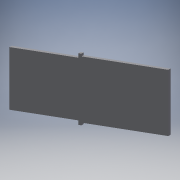
# Autodesk Inventor part: Zonnepaneel V5.0 print Versie
Saved by Autodesk Inventor 2018.3 (Build 223284000, 284)
## iProperties
Created: 2020-11-27
Part Number: Zonnepaneel V5.0 print Versie
Material: Generic
Document SubType Name: Modeling
Designer: daanv
Density: 1 g/cm^3
Appearance: Default
Author: daanv
Autodesk Inventor part; units mm, degrees
ref_plane "YZ Plane" through (0, 0, 0) normal (1, 0, 0) x (0, 1, 0)
ref_plane "XZ Plane" through (0, 0, 0) normal (0, 1, 0) x (-1, 0, 0)
ref_plane "XY Plane" through (0, 0, 0) normal (0, 0, 1) x (1, 0, 0)
sketch "Sketch6" plane through (0, 0, 0) normal (0, 0, 1) x (1, 0, 0)
  line L0 (0, 0) -> (0, 3)
  line L1 (0, 3) -> (129.9038, 78)
  line L2 (129.9038, 78) -> (129.9038, 75)
  line L3 (129.9038, 75) -> (0, 0)
  dimension "d18" = 3
  dimension "d19" = 150
  dimension "d20" = 120
  dimension "d21" = 3
  constraints: 8 end point, 1 parallel, 1 vertical
  measures "d18" distance of L0.start L0.end
  measures "d19" distance of L0.end L1.end
  measures "d20" angle of L0 L1
  measures "d21" distance of L1.end L2.end
extrude "Extrusion6" add sketch "Sketch6" along normal blind 70
sketch "Sketch8" plane through (0, 0, 70) normal (0, 0, 1) x (1, 0, 0)
  line L0 (56.2917, 35.5) -> (56.2917, 32.5) projected
  line L1 (129.9038, 78) -> (0, 3) projected
  line L2 (56.2917, 32.5) -> (58.8897, 34)
  line L3 (129.9038, 75) -> (0, 0) projected
  line L4 (58.8897, 34) -> (58.8897, 37)
  line L5 (0, 3) -> (129.9038, 78) projected
  line L6 (56.2917, 35.5) -> (58.8897, 37)
  line L7 (56.2917, 35.5) -> (56.2917, 32.5)
  dimension "d27" = 3
  constraints: 8 end point, 2 point on line, 1 collinear, 1 parallel, 1 vertical
  measures "d27" distance of L0.end L2.end
extrude "Extrusion8" add sketch "Sketch8" along normal blind 5
sketch "Sketch9" plane through (0, 0, 70) normal (0, 0, 1) x (1, 0, 0)
  line L0 (58.8897, 37) -> (58.8897, 34) projected
  line L1 (58.8897, 34) -> (129.9038, 75) projected
  line L2 (129.9038, 75) -> (129.9038, 78) projected
  line L3 (129.9038, 78) -> (58.8897, 37) projected
  point P0 (0, 0)
extrude "Extrusion9" add sketch "Sketch9" along normal blind 2
sketch "Sketch10" plane through (0, 0, 0) normal (0, 0, -1) x (-1, 0, 0)
  line L0 (0, 3) -> (-129.9038, 78) projected
  line L1 (-129.9038, 75) -> (0, 0) projected
  line L2 (0, 3) -> (-56.2917, 35.5)
  line L3 (-56.2917, 35.5) -> (-58.8897, 37)
  line L4 (-58.8897, 37) -> (-58.8897, 34)
  line L5 (0, 0) -> (-56.2917, 32.5) projected
  line L6 (-58.8897, 34) -> (-56.2917, 32.5)
  line L7 (-56.2917, 35.5) -> (-56.2917, 32.5) projected
  line L8 (-56.2917, 32.5) -> (-56.2917, 35.5)
  point P0 (-64.9519, 37.5)
  dimension "d32" = 65
  dimension "d33" = 3
  constraints: 10 end point, 3 point on line, 2 collinear, 1 midpoint, 1 vertical
  measures "d32" distance of L0.start L2.end
  measures "d33" distance of L2.end L3.end
extrude "Extrusion10" add sketch "Sketch10" along normal blind 5
sketch "Sketch11" plane through (0, 0, 0) normal (0, 0, -1) x (-1, 0, 0)
  line L0 (-58.8897, 34) -> (-58.8897, 37) projected
  line L1 (0, 3) -> (-129.9038, 78) projected
  line L2 (-129.9038, 78) -> (-129.9038, 75) projected
  line L3 (-129.9038, 75) -> (0, 0) projected
extrude "Extrusion11" add sketch "Sketch11" along normal blind 2
body "Solid2"
